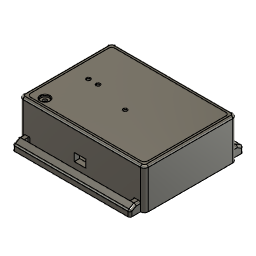
V4.0 Open-Source (Autodesk Fusion 360 design; units mm, degrees)
Autodesk Fusion 360 part; units mm, degrees
sketch "Top" plane through (0, 0, 0) normal (0, 1, 0) x (1, 0, 0)
  line L0 (35, -26.2) -> (48.95, -26.2) construction
  arc A0 (63, -48) -> (65, -46) centre (63, -46) ccw
  line L1 (63, -44) -> (63, -2)
  line L2 (38.05, -45.263) -> (25.05, -45.263)
  circle A1 centre (35, -26.2) radius 1.75
  line L3 (61.65, -14) -> (63, -14)
  line L4 (50.95, -35.25) -> (33, -35.25)
  line L5 (65, -2) -> (0, -2) construction
  circle A2 centre (35, -26.2) radius 1.4
  line L6 (39.475, -32.2956) -> (39.475, -27.2956)
  circle A3 centre (48.95, -26.2) radius 1.75
  line L7 (41.975, -26.2) -> (41.975, -27.2956) construction
  circle A4 centre (59.92, -22.92) radius 0.9 construction
  line L8 (58.127, -46) -> (58.127, -20.5)
  line L9 (25.05, -38.863) -> (38.05, -38.863) construction
  line L10 (30.3, -22) -> (33, -22)
  line L11 (2, 0) -> (63, 0)
  line L12 (2, -48) -> (63, -48)
  line L13 (39.55, -38.863) -> (39.55, -46) construction
  line L14 (3.35, -14) -> (2, -14)
  line L15 (29.5, -20.5) -> (29.5, -46) construction
  line L16 (2, -22) -> (30.3, -22) construction
  line L17 (63, -2) -> (2, -2)
  line L18 (63, -48) -> (63, 0) construction
  line L19 (61, -46) -> (4, -46)
  circle A5 centre (59.92, -43.58) radius 0.9 construction
  line L20 (25.05, -45.263) -> (25.05, -46)
  line L21 (50.95, -22) -> (58.127, -22)
  line L22 (38.05, -45.263) -> (38.05, -46)
  line L23 (38.05, -38.863) -> (39.55, -38.863) construction
  line L24 (33, -35.25) -> (33, -22)
  arc A6 (61, -46) -> (63, -44) centre (61, -44) ccw
  line L25 (2, -22) -> (0, -22) construction
  line L26 (2, -39.4) -> (30.3, -39.4)
  line L27 (30.3, -22) -> (30.3, -39.4)
  line L28 (2, -35.05) -> (25.085, -35.05)
  line L29 (39.475, -27.2956) -> (44.475, -27.2956)
  line L30 (44.475, -32.2956) -> (39.475, -32.2956)
  line L31 (2, -26.35) -> (25.085, -26.35)
  arc A7 (2, -44) -> (4, -46) centre (4, -44) ccw
  line L32 (33, -22) -> (50.95, -22)
  line L33 (65, -2) -> (65, -46)
  line L34 (0, -46) -> (0, -2)
  arc A8 (0, -46) -> (2, -48) centre (2, -46) ccw
  line L35 (38.05, -38.863) -> (38.05, -45.263) construction
  line L36 (25.085, -26.35) -> (25.085, -35.05)
  line L37 (6.88, -36.96) -> (6.88, -22) construction
  line L38 (25.05, -45.263) -> (25.05, -38.863) construction
  line L39 (23.55, -39.4) -> (23.55, -46)
  line L40 (0, -36.96) -> (6.88, -36.96) construction
  line L41 (2, -2) -> (2, -44)
  line L42 (8.127, -20.5) -> (8.127, -22)
  arc A9 (2, 0) -> (0, -2) centre (2, -2) ccw
  circle A10 centre (48.95, -26.2) radius 1.4
  line L43 (50.95, -22) -> (50.95, -35.25)
  line L44 (30.3, -39.4) -> (39.55, -39.4)
  arc A11 (65, -2) -> (63, 0) centre (63, -2) ccw
  line L45 (44.475, -27.2956) -> (44.475, -32.2956)
  line L46 (61.65, -17.5) -> (3.35, -17.5)
  line L47 (61.65, -14) -> (61.65, -2)
  line L48 (61.65, -17.5) -> (61.65, -14)
  line L49 (3.35, -14) -> (3.35, -2)
  line L50 (3.35, -17.5) -> (3.35, -14)
  line L51 (63, -19) -> (8.127, -19)
  line L52 (0, 0) -> (2, 0) construction
  line L53 (0, 0) -> (0, -2) construction
  line L54 (8.127, -20.5) -> (8.127, -19)
  circle A12 centre (8, -42.7) radius 2
  circle A13 centre (8, -42.7) radius 1
  line L55 (11.3, -46) -> (11.3, -39.4)
  line L56 (8.127, -22) -> (30.3, -22)
  line L57 (25.05, -39.4) -> (25.05, -45.263)
  line L58 (39.55, -39.4) -> (39.55, -46)
  line L59 (38.05, -39.4) -> (38.05, -45.263)
  line L60 (29.5, -20.5) -> (29.5, -22)
  line L61 (8.127, -20.5) -> (63, -20.5)
  line L62 (29.5, -22.6381) -> (36.034, -22.6381) construction
  line L63 (36.034, -22.6381) -> (36.9725, -20.5) construction
  line L64 (36.2, -20.5) -> (36.2, -22)
  point P0 (0, -48)
  point P1 (65, 0)
  dimension "d1" = 65
  dimension "d2" = 48
  dimension "d3" = 2
  dimension "d9" = 2
  dimension "d10" = 2
  dimension "d11" = 33.5
  dimension "d12" = 4.873
  dimension "d14" = 13.25
  dimension "d15" = 17.95
  dimension "d16" = 3.5
  dimension "d17" = 2
  dimension "d18" = 28.3
  dimension "d19" = 28.3
  dimension "d20" = 17.4
  dimension "d22" = 6.88
  dimension "d23" = 14.96
  dimension "d24" = 2
  dimension "d26" = 6.4
  dimension "d27" = 13
  dimension "d28" = 0.737
  dimension "d29" = 23.05
  dimension "d30" = 1.8
  dimension "d31" = 1.8
  dimension "d32" = 2.42
  dimension "d33" = 3.08
  dimension "d34" = 3.08
  dimension "d36" = 3.5
  dimension "d37" = 3.5
  dimension "d38" = 2
  dimension "d39" = 2
  dimension "d40" = 4.2
  dimension "d41" = 4.2
  dimension "d42" = 90
  dimension "d44" = 5
  dimension "d45" = 5
  dimension "d46" = 90
  dimension "d47" = 2.8
  dimension "d48" = 2.8
  dimension "d49" = 1.5
  dimension "d50" = 1.5
  dimension "d51" = 4.35
  dimension "d129" = 2
  dimension "d133" = 2.9544
  dimension "d134" = 4.35
  dimension "d135" = 5.215
  dimension "d139" = 0.537
  dimension "d140" = 1.35
  dimension "d141" = 1.35
  dimension "d142" = 15.5
  dimension "d143" = 1.5
  dimension "d146" = 2
  dimension "d147" = 50
  dimension "d148" = 12
  dimension "d149" = 12
  dimension "d163" = 4
  dimension "d164" = 3.3
  dimension "d165" = 6
  dimension "d166" = 2
  dimension "d167" = 3.3
  dimension "d208" = 25.5
  dimension "d266" = 6.534
  dimension "d267" = 113.7
  dimension "d268" = 2.335
  dimension "d269" = 6.7
  constraint vertical L33
  constraint coincident L52.start L53.start
  constraint coincident L5.start L33
  constraint coincident L5.end L34
  constraint perpendicular L5 L34
  constraint coincident L1.end L18
  constraint coincident L1.end L5
  constraint coincident L17.end L5
  constraint coincident L3.end L18
  constraint perpendicular L3 L18
  constraint perpendicular L12 L33
  constraint coincident A0.start L12
  constraint perpendicular L11 L33
  constraint coincident L18.end L11
  constraint coincident L52.start L34
  constraint coincident L52.start L11
  constraint tangent L34 A9
  constraint tangent L11 A9
  constraint coincident P0 L34
  constraint coincident P0 L12
  constraint tangent L34 A8
  constraint tangent L12 A8
  constraint equal A8 A9
  constraint tangent A0 L33
  constraint tangent A0 L12
  constraint equal A0 A9
  constraint coincident P1 L33
  constraint coincident P1 L11
  constraint tangent L33 A11
  constraint tangent L11 A11
  constraint equal A9 A11
  constraint coincident L15.end L19
  constraint perpendicular L15 L19
  constraint coincident L8.start L19
  constraint horizontal L32
  constraint vertical L43
  constraint horizontal L4
  constraint vertical L24
  constraint tangent A7 L41
  constraint tangent L19 A7
  constraint tangent L19 A6
  constraint tangent L1 A6
  constraint equal A6 A7
  constraint coincident L26.start L41
  constraint perpendicular L26 L41
  constraint coincident L40.start L34
  constraint perpendicular L34 L40
  constraint coincident L37.end L16
  constraint perpendicular L16 L37
  constraint coincident L25.end L34
  constraint perpendicular L25 L34
  constraint horizontal L9
  constraint vertical L35
  constraint horizontal L2
  constraint vertical L38
  constraint coincident L42.end L16
  constraint perpendicular L16 L42
  constraint parallel L10 L32
  constraint coincident L21.end L8
  constraint perpendicular L8 L21
  constraint horizontal L29
  constraint vertical L45
  constraint horizontal L30
  constraint vertical L6
  constraint coincident L0.start A1.centre
  constraint coincident L0.end A3.centre
  constraint midpoint L7.start L0
  constraint midpoint L7.end L29
  constraint concentric A1 A2
  constraint concentric A3 A10
  constraint coincident L22.end L19
  constraint perpendicular L19 L22
  constraint coincident L20.end L19
  constraint perpendicular L19 L20
  constraint perpendicular L20 L23
  constraint coincident L13.end L19
  constraint perpendicular L13 L19
  constraint coincident L39.start L26
  constraint coincident L39.end L19
  constraint perpendicular L19 L39
  constraint coincident L44.end L13
  constraint perpendicular L13 L44
  constraint coincident L14.end L41
  constraint coincident L31.start L41
  constraint perpendicular L31 L41
  constraint coincident L28.start L41
  constraint perpendicular L28 L37
  constraint perpendicular L28 L36
  constraint coincident L17 L47.end
  constraint perpendicular L3 L47
  constraint perpendicular L3 L48
  constraint coincident L17 L49.end
  constraint perpendicular L14 L49
  constraint perpendicular L14 L50
  constraint coincident L1 L51.start
  constraint perpendicular L41 L51
  constraint tangent A9 L52
  constraint concentric A12 A13
  constraint coincident L19 L55.start
  constraint coincident L26 L55.end
  constraint perpendicular L26 L55
  constraint coincident L26 L57.start
  constraint coincident L38 L57.start
  constraint coincident L35 L59.start
  constraint coincident L44 L59.start
  constraint coincident L16 L60.end
  constraint coincident L1 L61.end
  constraint coincident L8.end L61
  constraint coincident L15.start L61
  constraint perpendicular L1 L61
  constraint perpendicular L54 L61
  constraint perpendicular L60 L61
  constraint coincident L15 L62.start
  constraint perpendicular L24 L62
  constraint coincident L61 L63.end
  constraint coincident L61 L64.start
  constraint coincident L32 L64.end
  constraint perpendicular L32 L64
  measures "d1" distance of P1 L52.start
  measures "d2" distance of P0 L52.start
  measures "d3" distance of L18 L33
  measures "d9" radius of A9
  measures "d10" distance of L11 L17
  measures "d11" distance of L1 L15
  measures "d12" distance of L1 L8
  measures "d14" distance of L4 L32
  measures "d15" distance of L24 L43
  measures "d16" distance of L15 L24
  measures "d17" radius of A7
  measures "d18" distance of L26.start L26.end
  measures "d19" distance of L10.start L16.start
  measures "d20" distance of L16 L26
  measures "d22" distance of L37.start L40.start
  measures "d23" distance of L37.start L37.end
  measures "d24" distance of L34 L41
  measures "d26" distance of L2.end L9.start
  measures "d27" distance of L35 L38
  measures "d28" distance of L2 L19
  measures "d29" distance of L38 L41
  measures "d30" diameter of A5
  measures "d31" diameter of A4
  measures "d32" distance of A5.centre L19
  measures "d33" distance of A5.centre L1
  measures "d34" distance of A4.centre L18
  measures "d36" diameter of A1
  measures "d37" diameter of A3
  measures "d38" distance of L0.end L43
  measures "d39" distance of L0.start L24
  measures "d40" distance of L0.start L32
  measures "d41" distance of L0.end L32
  measures "d42" angle of L10 L27
  measures "d44" distance of L30.start L29.end
  measures "d45" distance of L6 L45
  measures "d46" angle of L0 L7
  measures "d47" diameter of A2
  measures "d48" diameter of A10
  measures "d49" distance of L9.end L13.start
  measures "d50" distance of L38 L39
  measures "d51" distance of L26 L28
  measures "d129" distance of L12 L19
  measures "d133" distance of L4 L30
  measures "d134" distance of L16 L31
  measures "d135" distance of L27 L36
  measures "d139" distance of L9 L26
  measures "d140" distance of L1 L47
  measures "d141" distance of L41 L49
  measures "d142" distance of L17 L46
  measures "d143" distance of L46 L51
  measures "d146" distance of L11.start L52.start
  measures "d147" distance of L8 L42
  measures "d148" distance of L14 L17
  measures "d149" distance of L3 L17
  measures "d163" diameter of A12
  measures "d164" distance of L19 A12.centre
  measures "d165" distance of L41 A12.centre
  measures "d166" diameter of A13
  measures "d167" distance of A12.centre L55
  measures "d208" distance of L19 L61
  measures "d266" distance of L62.start L62.end
  measures "d267" angle of L61 L63
  measures "d268" distance of L62.end L63.end
  measures "d269" distance of L60 L64
sketch "TP4056+JST" plane through (0, 0, 0) normal (1, 0, 0) x (0, 0, -1)
  line L0 (-22, 4.5) -> (-39.4, 4.5) construction
  line L1 (-26.4, 5.78) -> (-26.4, 5.86)
  arc A0 (-33.87, 8.205) -> (-35.87, 6.205) centre (-33.87, 6.205) ccw
  line L2 (-25.53, 5.435) -> (-35.87, 5.435)
  line L3 (-25.53, 5.435) -> (-25.53, 6.205)
  arc A1 (-35.87, 5.435) -> (-33.87, 3.435) centre (-33.87, 5.435) ccw
  arc A2 (-35, 5.78) -> (-33.65, 4.43) centre (-33.65, 5.78) ccw
  line L4 (-22, 3) -> (-22, 4.5) construction
  line L5 (-27.75, 7.21) -> (-33.65, 7.21)
  arc A3 (-27.75, 4.43) -> (-26.4, 5.78) centre (-27.75, 5.78) ccw
  arc A4 (-27.53, 3.435) -> (-25.53, 5.435) centre (-27.53, 5.435) ccw
  line L6 (-39.4, 4.5) -> (-39.4, 3) construction
  arc A5 (-25.53, 6.205) -> (-27.53, 8.205) centre (-27.53, 6.205) ccw
  line L7 (-33.87, 3.435) -> (-27.53, 3.435)
  line L8 (-35.87, 5.435) -> (-37.96, 5.435)
  line L9 (-37.96, 5.435) -> (-37.96, 10.435)
  line L10 (-35, 5.86) -> (-35, 5.78)
  line L11 (-33.65, 4.43) -> (-27.75, 4.43)
  line L12 (-30.7, 3) -> (-30.7, 7.21) construction
  line L13 (-25.53, 5.435) -> (-23.44, 5.435)
  line L14 (-27.53, 8.205) -> (-33.87, 8.205)
  arc A6 (-33.65, 7.21) -> (-35, 5.86) centre (-33.65, 5.86) ccw
  line L15 (-35.87, 6.205) -> (-35.87, 5.435)
  arc A7 (-26.4, 5.86) -> (-27.75, 7.21) centre (-27.75, 5.86) ccw
  line L16 (-23.44, 5.435) -> (-23.44, 10.435)
  line L17 (-39.4, 3) -> (-22, 3) construction
  line L18 (0, 0) -> (-48, 0)
  line L19 (-48, 0) -> (-48, 21)
  line L20 (-48, 21) -> (0, 21)
  line L21 (0, 21) -> (0, 0)
  line L22 (-23.44, 10.435) -> (-37.96, 10.435)
  line L23 (-44, 6) -> (-44, 7)
  line L24 (-43, 5) -> (-42, 5)
  line L25 (-41, 6) -> (-41, 7)
  line L26 (-42, 8) -> (-43, 8)
  arc A8 (-41, 7) -> (-42, 8) centre (-42, 7) ccw
  arc A9 (-43, 8) -> (-44, 7) centre (-43, 7) ccw
  arc A10 (-44, 6) -> (-43, 5) centre (-43, 6) ccw
  arc A11 (-42, 5) -> (-41, 6) centre (-42, 6) ccw
  point P0 (-26.4, 7.21)
  point P1 (-26.4, 4.43)
  point P2 (-35, 7.21)
  point P3 (-35.87, 8.205)
  point P4 (-25.53, 8.205)
  point P5 (-25.53, 3.435)
  point P6 (-44, 5)
  dimension "d58" = 1.5
  dimension "d59" = 17.4
  dimension "d62" = 8.6
  dimension "d63" = 2.78
  dimension "d64" = 1.43
  dimension "d65" = 90
  dimension "d66" = 1.35
  dimension "d67" = 10.34
  dimension "d68" = 4.77
  dimension "d69" = 5.17
  dimension "d70" = 0.995
  dimension "d71" = 2
  dimension "d76" = 2.09
  dimension "d150" = 48
  dimension "d151" = 21
  dimension "d153" = 3.435
  dimension "d155" = 0.87
  dimension "d206" = 30.7
  dimension "d330" = 2.09
  dimension "d331" = 5
  dimension "d341" = 4
  dimension "d342" = 5
  dimension "d343" = 3
  dimension "d344" = 3
  dimension "d345" = 1
  constraint horizontal L0
  constraint vertical L6
  constraint horizontal L17
  constraint vertical L4
  constraint horizontal L5
  constraint vertical L10
  constraint horizontal L11
  constraint vertical L1
  constraint midpoint L12.start L17
  constraint coincident L12.end L5
  constraint coincident P0 L5
  constraint coincident P0 L1
  constraint tangent L5 A7
  constraint tangent L1 A7
  constraint coincident P2 L5
  constraint coincident P2 L10
  constraint tangent L5 A6
  constraint tangent L10 A6
  constraint equal A6 A7
  constraint tangent A2 L10
  constraint tangent A2 L11
  constraint equal A2 A7
  constraint coincident P1 L11
  constraint coincident P1 L1
  constraint tangent A3 L11
  constraint tangent L1 A3
  constraint equal A3 A7
  constraint horizontal L14
  constraint vertical L15
  constraint horizontal L7
  constraint vertical L3
  constraint coincident P4 L14
  constraint coincident P4 L3
  constraint tangent A5 L14
  constraint tangent L3 A5
  constraint coincident P3 L14
  constraint coincident P3 L15
  constraint tangent A0 L14
  constraint tangent A0 L15
  constraint equal A0 A5
  constraint tangent A1 L15
  constraint tangent A1 L7
  constraint equal A1 A5
  constraint coincident P5 L7
  constraint coincident P5 L3
  constraint tangent A4 L7
  constraint tangent L3 A4
  constraint equal A4 A5
  constraint perpendicular L3 L13
  constraint horizontal L18
  constraint vertical L19
  constraint horizontal L20
  constraint vertical L21
  constraint coincident L18.start L21.end
  constraint perpendicular L8 L9
  constraint horizontal L22
  constraint coincident L16.end L22.start
  constraint perpendicular L16 L22
  constraint coincident L9.end L22.end
  constraint vertical L23
  constraint perpendicular L23 L24
  constraint perpendicular L24 L25
  constraint perpendicular L25 L26
  constraint tangent L25 A8
  constraint tangent L26 A8
  constraint tangent L23 A9
  constraint tangent L26 A9
  constraint equal A8 A9
  constraint coincident P6 L23
  constraint coincident P6 L24
  constraint tangent L23 A10
  constraint tangent L24 A10
  constraint equal A8 A10
  constraint tangent L24 A11
  constraint tangent L25 A11
  constraint equal A8 A11
  measures "d58" distance of L0 L17
  measures "d59" distance of L6.end L4.start
  measures "d62" distance of P0 P2
  measures "d63" distance of P0 P1
  measures "d64" distance of L11 L17
  measures "d65" angle of L12 L17
  measures "d66" radius of A7
  measures "d67" distance of P3 P4
  measures "d68" distance of P4 P5
  measures "d69" distance of L3 L12
  measures "d70" distance of L5 L14
  measures "d71" radius of A5
  measures "d76" distance of L2.start L13.end
  measures "d150" distance of L18.start L18.end
  measures "d151" distance of L18.start L20.end
  measures "d153" distance of L7 L18
  measures "d155" distance of L1 L3
  measures "d206" distance of L12 L21
  measures "d330" distance of L9 L15
  measures "d331" distance of L13.end L16.end
  measures "d341" distance of L19 L23
  measures "d342" distance of L18 P6
  measures "d343" distance of L23 L25
  measures "d344" distance of L24 L26
  measures "d345" radius of A8
ref_plane "WorkPlane2" through (0, 19, 0) normal (0, 1, 0) x (0, 0, 1)
sketch "Lid" plane through (0, 19, 0) normal (0, 1, 0) x (1, 0, 0)
  line L0 (0, 0) -> (65, 0) construction
  line L1 (65, 0) -> (65, -48) construction
  line L2 (65, -48) -> (0, -48) construction
  line L3 (0, -48) -> (0, 0) construction
  line L4 (63, -3.5) -> (63, -44)
  line L5 (61, -46) -> (4, -46)
  line L6 (2, -44) -> (2, -3.5)
  line L7 (3.5, -2) -> (61.5, -2)
  arc A0 (2, -44) -> (4, -46) centre (4, -44) ccw
  arc A1 (61, -46) -> (63, -44) centre (61, -44) ccw
  line L8 (2, -39.4) -> (30.3, -39.4) construction
  line L9 (30.3, -39.4) -> (30.3, -22) construction
  line L10 (30.3, -22) -> (2, -22) construction
  line L11 (28.3, -39.4) -> (28.3, -22) construction
  line L12 (63, -20.5) -> (36.973, -20.5) construction
  line L13 (58.127, -46) -> (58.127, -20.5) construction
  line L14 (36.973, -20.5) -> (36.1657, -22.339) construction
  line L15 (35.7079, -22.6381) -> (30.0005, -22.6381) construction
  arc A2 (35.7079, -22.6381) -> (36.1657, -22.339) centre (35.7079, -22.1381) ccw construction
  line L16 (29.5005, -23.1381) -> (29.5005, -46) construction
  arc A3 (30.0005, -22.6381) -> (29.5005, -23.1381) centre (30.0005, -23.1381) ccw construction
  line L17 (32.5005, -37.82) -> (29.5005, -37.82)
  line L18 (32.5005, -37.82) -> (32.5005, -39.82)
  line L19 (32.5005, -39.82) -> (29.5005, -39.82)
  line L20 (29.5005, -39.82) -> (29.5005, -37.82)
  line L21 (32.5005, -37.82) -> (32.5005, -28.68)
  line L22 (26.9005, -28.2) -> (29.3005, -28.2)
  line L23 (29.3005, -28.2) -> (29.3005, -33.2)
  line L24 (29.3005, -33.2) -> (26.9005, -33.2)
  line L25 (26.9005, -33.2) -> (26.9005, -28.2)
  line L26 (32.5005, -28.68) -> (29.5005, -28.68)
  line L27 (32.5005, -26.68) -> (29.5005, -26.68)
  line L28 (28.4005, -33.2) -> (28.4005, -28.2)
  line L29 (29.3005, -33.2) -> (29.5005, -33.2)
  line L30 (29.3005, -28.2) -> (29.5005, -28.2)
  line L31 (29.5005, -26.68) -> (29.5005, -28.2)
  line L32 (29.5005, -33.2) -> (29.5005, -37.82)
  line L33 (29.5005, -28.68) -> (29.5005, -28.2)
  circle A4 centre (34.076, -27.053) radius 0.75
  line L34 (32.5005, -28.68) -> (32.5005, -26.68)
  circle A5 centre (10.65, -22.7) radius 0.75
  circle A6 centre (15.65, -22.7) radius 0.75
  circle A7 centre (8, -42.7) radius 2.25
  line L35 (11.3, -46) -> (11.3, -39.4)
  line L36 (11.3, -39.4) -> (2, -39.4)
  line L37 (58.127, -46) -> (58.127, -20.5)
  line L38 (63, -20.5) -> (58.127, -20.5)
  circle A8 centre (8, -42.7) radius 1
  arc A9 (3.5, -2) -> (2, -3.5) centre (3.5, -3.5) ccw
  arc A10 (63, -3.5) -> (61.5, -2) centre (61.5, -3.5) ccw
  line L39 (60, -45) -> (58.127, -45)
  arc A11 (60, -45) -> (62, -43) centre (60, -43) ccw
  line L40 (62, -43) -> (62, -21.5)
  line L41 (62, -21.5) -> (58.127, -21.5)
  point P0 (36.0345, -22.6381)
  point P1 (29.5005, -22.6381)
  dimension "d98" = 65
  dimension "d99" = 48
  dimension "d101" = 2
  dimension "d102" = 6.6
  dimension "d103" = 28.3
  dimension "d104" = 17.4
  dimension "d105" = 2
  dimension "d106" = 25.5
  dimension "d107" = 4.873
  dimension "d109" = 26.027
  dimension "d110" = 113.7
  dimension "d112" = 6.534
  dimension "d113" = 2.335
  dimension "d114" = 0.5
  dimension "d115" = 0.5
  dimension "d116" = 8.18
  dimension "d117" = 2
  dimension "d121" = 6.2
  dimension "d122" = 5
  dimension "d123" = 2
  dimension "d124" = 9.14
  dimension "d125" = 0.2
  dimension "d126" = 2.4
  dimension "d127" = 1.5
  dimension "d128" = 3
  dimension "d171" = 1.5
  dimension "d172" = 18.947
  dimension "d173" = 28.924
  dimension "d174" = 1.5
  dimension "d175" = 1.5
  dimension "d176" = 8.65
  dimension "d177" = 23.3
  dimension "d178" = 5
  dimension "d179" = 4.5
  dimension "d181" = 3.3
  dimension "d182" = 6
  dimension "d183" = 3.3
  dimension "d231" = 2
  dimension "d316" = 1.5
  dimension "d317" = 2
  dimension "d318" = 1
  dimension "d320" = 1
  dimension "d321" = 1
  constraint horizontal L0
  constraint vertical L1
  constraint horizontal L2
  constraint vertical L3
  constraint coincident L0.start L3.end
  constraint tangent L5 A0
  constraint tangent L6 A0
  constraint tangent L4 A1
  constraint tangent L5 A1
  constraint equal A0 A1
  constraint coincident L6 L8.start
  constraint perpendicular L6 L8
  constraint perpendicular L8 L9
  constraint coincident L6 L10.end
  constraint perpendicular L6 L10
  constraint coincident L8 L11.start
  constraint coincident L10 L11.end
  constraint perpendicular L10 L11
  constraint coincident L4 L12.start
  constraint perpendicular L4 L12
  constraint coincident L5 L13.start
  constraint coincident L12 L13.end
  constraint perpendicular L12 L13
  constraint horizontal L15
  constraint coincident P0 L14
  constraint coincident P0 L15
  constraint tangent L14 A2
  constraint tangent L15 A2
  constraint coincident L5 L16.end
  constraint perpendicular L5 L16
  constraint coincident P1 L15
  constraint coincident P1 L16
  constraint tangent L15 A3
  constraint tangent L16 A3
  constraint perpendicular L16 L17
  constraint perpendicular L17 L18
  constraint perpendicular L16 L19
  constraint perpendicular L17 L20
  constraint perpendicular L17 L21
  constraint perpendicular L11 L22
  constraint perpendicular L22 L23
  constraint perpendicular L23 L24
  constraint perpendicular L22 L25
  constraint coincident L16 L26.end
  constraint perpendicular L16 L26
  constraint coincident L16 L27.end
  constraint perpendicular L16 L27
  constraint coincident L24 L28.start
  constraint coincident L22 L28.end
  constraint perpendicular L22 L28
  constraint coincident L16 L29.end
  constraint perpendicular L16 L29
  constraint coincident L16 L30.end
  constraint perpendicular L16 L30
  constraint perpendicular L17 L32
  constraint perpendicular L27 L34
  constraint horizontal A5.centre A6.centre
  constraint coincident L5 L35.start
  constraint coincident L8 L35.end
  constraint perpendicular L8 L35
  constraint concentric A7 A8
  constraint tangent L6 A9
  constraint tangent L7 A9
  constraint tangent L4 A10
  constraint tangent L7 A10
  constraint equal A9 A10
  constraint coincident L37 L39.end
  constraint perpendicular L37 L39
  constraint tangent L39 A11
  constraint tangent A11 L40
  constraint parallel L37 L40
  constraint coincident L13 L41.end
  constraint perpendicular L13 L41
  measures "d98" distance of L0.start L0.end
  measures "d99" distance of L0.start L2.end
  measures "d101" radius of A0
  measures "d102" distance of L5 L8
  measures "d103" distance of L8.start L8.end
  measures "d104" distance of L8.end L9.end
  measures "d105" distance of L9 L11
  measures "d106" distance of L5 L12
  measures "d107" distance of L4 L13
  measures "d109" distance of L4 L12.end
  measures "d110" angle of L12 L14
  measures "d112" distance of P0 P1
  measures "d113" distance of L12.end P0
  measures "d114" radius of A2
  measures "d115" radius of A3
  measures "d116" distance of L5 L17
  measures "d117" distance of L17.start L18.end
  measures "d121" distance of L8 L24
  measures "d122" distance of L22 L24
  measures "d123" distance of L26 L27
  measures "d124" distance of L17 L26
  measures "d125" distance of L16 L23
  measures "d126" distance of L22.start L22.end
  measures "d127" distance of L25 L28
  measures "d128" distance of L16 L21
  measures "d171" diameter of A4
  measures "d172" distance of L5 A4.centre
  measures "d173" distance of L4 A4.centre
  measures "d174" diameter of A5
  measures "d175" diameter of A6
  measures "d176" distance of L6 A5.centre
  measures "d177" distance of L5 A5.centre
  measures "d178" distance of A5.centre A6.centre
  measures "d179" diameter of A7
  measures "d181" distance of L5 A7.centre
  measures "d182" distance of L6 A7.centre
  measures "d183" distance of A7.centre L35
  measures "d231" diameter of A8
  measures "d316" radius of A9
  measures "d317" radius of A11
  measures "d318" distance of L5 L39
  measures "d320" distance of L38 L41
  measures "d321" distance of L4 L40
extrude "Extrude10" add sketch "Top" along normal blind 1.5 contours L1 L3 L14 L26 L27 L28 L31 L36 L41 L42 L46 L48 L50 L51 L54 L56 | L4 L24 L32 L43 makes body 1 at (28.5617, 0, 32.15) makes body 2 at (48.0814, 0, 31.8302)
extrude "Extrude11" add sketch "Top" along normal blind 3 contours L17 L46 L47 L48 L49 L50 | L28 L31 L36 L41 | A1 | L6 L29 L30 L45 | A3 bodies 1 2
extrude "Extrude12" add sketch "Top" along normal blind 5 contours L4 L8 L10 L19 L21 L24 L27 L43 L44 L58 | L42 L56 L60 L61 | L2 L26 L44 L57 L59 | L19 L26 L39 L55 bodies 1 2
extrude "Extrude13" add sketch "Top" along normal blind 10.85 contours L1 L8 L19 A6 L61 | L8 L21 L32 L61 L64 | L10 L32 L56 L60 L61 L64 | L19 L22 L44 L58 L59 | L2 L19 L20 L22 | L19 L20 L26 L39 L57 | A2 | A10 bodies 1
extrude "Extrude16" add sketch "Top" along normal blind 21 contours A0 L11 L12 L33 L34 A8 A9 A11 bodies 1
extrude "Extrude20" add sketch "Lid" against normal blind 17.5 separate body contours L22 L23 L24 L28 makes body 3
extrude "Extrude21" add sketch "Lid" against normal blind 14.5 contours L22 L24 L25 L28 bodies 3
extrude "Extrude22" add sketch "Lid" against normal blind 4 contours L17 L21 L23 L26 L29 L30 L32 L33 bodies 3
extrude "Extrude23" add sketch "Lid" against normal blind 7.15 contours L17 L18 L19 L20 | L26 L27 L31 L33 L34 bodies 3
chamfer "Chamfer2" distance 0.5 angle 45 2 edges at (33.6947, 10.85, 26.7063) (47.6447, 10.85, 26.7063) on bodies 1
sketch "Switch" plane through (0, 0, 46) normal (0, 0, -1) x (-1, 0, 0)
  line L0 (-61, 10.85) -> (-58.127, 10.85)
  line L1 (-58.127, 10.85) -> (-58.127, 5)
  line L2 (-58.127, 5) -> (-39.55, 5)
  line L3 (-39.55, 5) -> (-39.55, 10.85)
  line L4 (-39.55, 10.85) -> (-23.55, 10.85)
  line L5 (-23.55, 10.85) -> (-23.55, 5)
  line L6 (-4, 0) -> (-4, 21)
  line L7 (-4, 21) -> (-61, 21)
  line L8 (-61, 21) -> (-61, 10.85)
  line L9 (-23.55, 5) -> (-39.55, 5)
  line L10 (-25.05, 5) -> (-25.05, 10.85)
  line L11 (-38.05, 5) -> (-38.05, 5.3288)
  line L12 (-38.05, 5.3288) -> (-38.05, 10.85)
  line L13 (-23.55, 5) -> (-23.55, 10.85)
  line L14 (-25.05, 10.85) -> (-23.55, 10.85)
  line L15 (-39.55, 5) -> (-39.55, 10.85)
  line L16 (-38.05, 10.85) -> (-39.55, 10.85)
  line L17 (-38.05, 10.85) -> (-25.05, 10.85)
  line L18 (-34.55, 9.515) -> (-28.55, 9.515)
  line L19 (-28.55, 9.515) -> (-28.55, 5.415)
  line L20 (-28.55, 5.415) -> (-34.55, 5.415)
  line L21 (-34.55, 5.415) -> (-34.55, 9.515)
  line L22 (-23.55, 10.85) -> (-23.55, 19)
  line L23 (-23.55, 19) -> (-25.05, 19)
  line L24 (-25.05, 19) -> (-25.05, 10.85)
  line L25 (0, 0) -> (-32.2604, 0) construction
  line L26 (0, 0) -> (0, 23.5045) construction
  line L27 (-29.5, 10.85) -> (-29.5, 19)
  line L28 (-29.5, 19) -> (-25.05, 19)
  line L29 (-23.55, 5) -> (-11.3, 5)
  line L30 (-11.3, 5) -> (-11.3, 0)
  line L31 (-11.3, 0) -> (-4, 0)
  dimension "d250" = 1.5
  dimension "d251" = 1.5
  dimension "d252" = 3.5
  dimension "d253" = 0.415
  dimension "d254" = 6
  dimension "d255" = 4.1
  dimension "d256" = 19
  dimension "d263" = 29.5
  constraint coincident L5.end L9.start
  constraint coincident L2.end L3.start
  constraint coincident L9 L10.start
  constraint coincident L4 L10.end
  constraint perpendicular L4 L10
  constraint coincident L9 L11.start
  constraint perpendicular L9 L11
  constraint coincident L4 L12.end
  constraint perpendicular L4 L12
  constraint coincident L4.end L5.start
  constraint coincident L3.end L4.start
  constraint horizontal L18
  constraint vertical L19
  constraint horizontal L20
  constraint vertical L21
  constraint perpendicular L4 L22
  constraint perpendicular L10 L23
  constraint perpendicular L4 L24
  constraint coincident L25.start L26.start
  constraint horizontal L25
  constraint perpendicular L25 L26
  constraint coincident L17 L27.start
  constraint perpendicular L17 L27
  constraint perpendicular L27 L28
  measures "d250" distance of L3 L12
  measures "d251" distance of L5 L10
  measures "d252" distance of L10 L19
  measures "d253" distance of L9 L20
  measures "d254" distance of L19 L21
  measures "d255" distance of L18 L20
  measures "d256" distance of L23 L25
  measures "d263" distance of L26 L27
extrude "Extrude27" cut sketch "Switch" along normal blind 0.737 and the other way blind 2 contours L18 L19 L20 L21 bodies 1
extrude "Extrude28" add sketch "Switch" along normal blind 6.6 contours L4 L14 L22 L23 L24 bodies 1
extrude "Extrude29" add sketch "Switch" along normal blind 0.737 contours L4 L17 L24 L27 L28 bodies 1
extrude "Extrude30" add sketch "Top" along normal blind 19 contours L10 L32 L56 L60 L61 L64 bodies 1
fillet "Fillet3" radius 1 8 edges at (32.5, 21, 48) (64.4142, 21, 47.4142) (65, 21, 24) (64.4142, 21, 0.5858) (32.5, 21, 0) (0.5858, 21, 0.5858) (0, 21, 24) (0.5858, 21, 47.4142) on bodies 1
sketch "Strap Loop" plane through (0, 0, 0) normal (-1, 0, 0) x (0, 0, 1)
  line L0 (46, 20) -> (2, 20)
  line L1 (2, 20) -> (2, 0)
  line L2 (2, 0) -> (46, 0)
  line L3 (46, 0) -> (46, 20)
  line L4 (0, 0) -> (48, 0)
  line L5 (48, 0) -> (48, 21)
  line L6 (48, 21) -> (0, 21)
  line L7 (0, 21) -> (0, 0)
  line L8 (48, 0) -> (50.5, 0)
  line L9 (50.5, 0) -> (53.5, 0)
  line L10 (53.5, 0) -> (53.5, 3)
  line L11 (50.5, 0) -> (50.5, 4.7321)
  line L12 (53.5, 3) -> (50.5, 4.7321)
  line L13 (50.5, 4.7321) -> (48, 4.7321)
  line L14 (24, 0) -> (24, 21) construction
  line L15 (0, 0) -> (-2.5, 0)
  line L16 (-5.5, 0) -> (-5.5, 3)
  line L17 (-5.5, 3) -> (-2.5, 4.7321)
  line L18 (-2.5, 0) -> (-5.5, 0)
  line L19 (-2.5, 0) -> (-2.5, 4.7321)
  line L20 (-2.5, 4.7321) -> (0, 4.7321)
  dimension "d283" = 48
  dimension "d284" = 21
  dimension "d285" = 2.5
  dimension "d286" = 3
  dimension "d287" = 3
  dimension "d289" = 120
  constraint horizontal L4
  constraint vertical L5
  constraint horizontal L6
  constraint vertical L7
  constraint coincident L4.start L7.end
  constraint perpendicular L5 L8
  constraint parallel L8 L9
  constraint perpendicular L9 L10
  constraint perpendicular L8 L11
  constraint coincident L5 L13.end
  constraint perpendicular L5 L13
  constraint midpoint L4 L14.start
  constraint midpoint L6 L14.end
  constraint coincident L4.end L5.start
  constraint symmetric L4.end L14 L4.start
  constraint symmetric L8.end L14 L15.end
  constraint symmetric L9.end L14 L16.start
  constraint symmetric L10.end L14 L16.end
  constraint symmetric L11.end L14 L17.end
  constraint symmetric L13.end L14 L20.end
  measures "d283" distance of L4.start L4.end
  measures "d284" distance of L4.start L6.end
  measures "d285" distance of L4.end L8.end
  measures "d286" distance of L8.end L9.end
  measures "d287" distance of L9.end L10.end
  measures "d289" angle of L10 L12
extrude "Extrude31" add sketch "Strap Loop" along normal blind -2 and the other way blind 63 separate body contours L9 L10 L11 L12 | L16 L17 L18 L19 makes body 4 at (42.6667, 1.5774, 50.5) makes body 5 at (22.3333, 1.5774, -2.5)
extrude "Extrude32" add sketch "Strap Loop" along normal blind -2 and the other way blind 5 contours L5 L8 L11 L13 | L7 L15 L19 L20 | L9 L10 L11 L12 | L16 L17 L18 L19 bodies 4 1 5
extrude "Extrude33" add sketch "Strap Loop" along normal blind -60 and the other way blind 63 contours L5 L8 L11 L13 | L7 L15 L19 L20 | L9 L10 L11 L12 | L16 L17 L18 L19 bodies 4
extrude "Extrude34" add sketch "Lid" against normal blind 7.15 separate body contours L37 L39 A11 L40 L41 makes body 6
extrude "Extrude35" add sketch "Lid" along normal blind 2 contours L4 L5 L6 L7 L35 L36 L37 L38 A9 A10 | L4 L5 A1 L37 L38 L39 A11 L40 L41 | L37 L39 A11 L40 L41 | L5 L6 A0 L35 L36 | L17 L18 L19 L20 | L17 L21 L23 L26 L29 L30 L32 L33 | L26 L27 L31 L33 L34 | L22 L23 L24 L28 | L22 L24 L25 L28 bodies 3 6
extrude "Extrude36" add sketch "Lid" along normal blind 1 contours A7 bodies 3
fillet "Fillet11" radius 0.3 4 edges at (14.9508, 21, 22.4288) (9.9508, 21, 22.4288) (33.3768, 21, 26.7818) (5.9023, 21, 41.8864) on bodies 3
extrude "Extrude37" add sketch "Top" along normal blind 5 contours L19 L26 A7 L41 L55 bodies 4
extrude "Extrude38" add sketch "Top" along normal blind 19 contours L1 L51 L54 L61 | L1 L3 L17 L47 | L14 L17 L41 L49 | A12 bodies 4
extrude "Extrude39" add sketch "Top" along normal blind 10 contours A13 bodies 4
fillet "Fillet12" radius 1.5 2 edges at (63, 20, 2) (2, 20, 2) on bodies 4
extrude "Extrude40" cut sketch "TP4056+JST" along normal blind 2 contours L1 L2 A2 L5 A3 L10 A6 A7 | L1 A0 L2 L3 A2 L5 A3 A5 L10 L14 A6 L15 A7 | L2 A2 A3 L11 | L2 A1 A2 A3 A4 L7 L11 | L23 L24 L25 L26 A8 A9 A10 A11 bodies 4
extrude "Extrude41" add sketch "TP4056+JST" along normal blind 3 and the other way blind -2 contours L1 A0 L2 L3 A2 L5 A3 A5 L10 L14 A6 L15 A7 | A0 L3 A5 L8 L9 L13 L14 L15 L16 L22 bodies 4
chamfer "Chamfer4" distance 1 angle 45 7 edges at (3, 7.21, 30.7) (3, 6.8146, 26.7954) (3, 5.82, 26.4) (3, 5.606, 26.4113) (3, 5.606, 34.9887) (3, 5.82, 35) (3, 6.8146, 34.6046) on bodies 4
fillet "Fillet13" radius 0.5 8 edges at (60, 2.366, 0) (60, 2.366, -2.5) (5, 2.366, 0) (5, 2.366, -2.5) (5, 2.366, 48) (5, 2.366, 50.5) (60, 2.366, 50.5) (60, 2.366, 48) on bodies 4
fillet "Fillet14" radius 1 4 edges at (63, 1.5, 53.5) (2, 1.5, 53.5) (2, 1.5, -5.5) (63, 1.5, -5.5) on bodies 4
fillet "Fillet15" radius 1 14 edges at (2, 4.1547, -3.5) (2.2929, 3.1691, -5.2071) (32.5, 3, -5.5) (62.7071, 3.1691, -5.2071) (63, 4.1547, -3.5) (2, 4.1547, 51.5) (2.2929, 3.1691, 53.2071) (32.5, 3, 53.5) (62.7071, 3.1691, 53.2071) (63, 4.1547, 51.5) (63, 4.7321, 49.25) (2, 4.7321, 49.25) (2, 4.7321, -1.25) (63, 4.7321, -1.25) on bodies 4
named bodies: "Case Body", "Lid"
